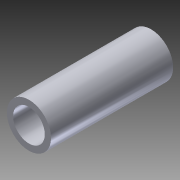
# Autodesk Inventor part: 0.75 Pipe
Saved by Autodesk Inventor 2013 (Build 170138000, 138)
## iProperties
Created: 2014-07-04
Part Number: 0.75 Pipe
Material: PVC-Piping
Document SubType Name: Modeling
Designer: Kyle
Density: 1 g/cm^3
Author: Kyle
Autodesk Inventor part; units mm, degrees
ref_plane "YZ Plane" through (0, 0, 0) normal (1, 0, 0) x (0, 1, 0)
ref_plane "XZ Plane" through (0, 0, 0) normal (0, 1, 0) x (-1, 0, 0)
ref_plane "XY Plane" through (0, 0, 0) normal (0, 0, 1) x (1, 0, 0)
sketch "Sketch1" plane through (0, 0, 0) normal (0, 0, 1) x (1, 0, 0)
  circle A0 centre (0, 0) radius 7.747
  circle A1 centre (0, 0) radius 10.795
  dimension "d0" = 21.59
  dimension "d2" = 15.494
  constraints: 2 centre point, 2 coincident
  measures "d0" diameter of A1
  measures "d2" diameter of A0
extrude "Extrusion1" add sketch "Sketch1" along normal blind 59.69
body "Solid1"
